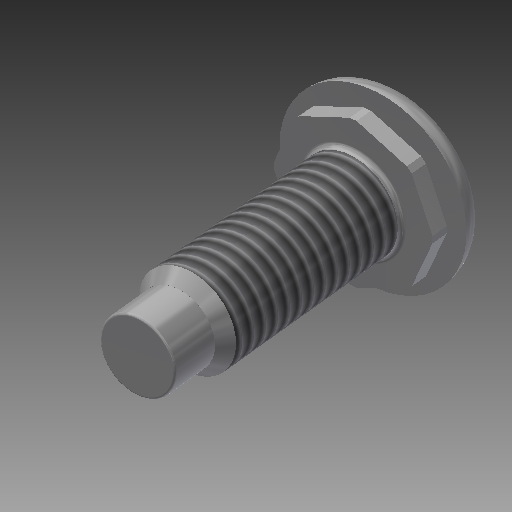
# Autodesk Inventor part: 314-10
Saved by Autodesk Inventor 2019 (Build 230136000, 136)
## iProperties
Company: Autodesk Inc.
Created: 2007-10-17
Part Number: 314-10
Document SubType Name: Modeling
Designer: Autodesk Inc.
Density: 7.85 g/cm^3
Mass: 23.0419 g
Surface Area: 17.262 cm^2
Volume: 2.93528 cm^3
Material: Steel, Mild
Description: DR342 M12 X 14
Appearance: Steel
Component Category: Fasteners
Author: Inventor
Autodesk Inventor part; units mm, degrees
ref_plane "YZ Plane" through (0, 0, 0) normal (1, 0, 0) x (0, 1, 0)
ref_plane "Work Plane1" through (2733.5993, 510.3823, 544.9206) normal (0.1045285, 0, 0.9945219) x (0.0000001, 1, 0)
sketch "Sketch1" plane through (2733.5993, 510.3823, 544.9206) normal (0.1045285, 0, 0.9945219) x (0.0000001, 1, 0)
  circle A0 centre (0, 3.6) radius 3.85
  line L0 (-510.3825, -1.79) -> (-510.3825, 8.99) projected
  line L1 (-5.3902, 2661.6646) -> (5.3898, 2661.6646) projected
  line L2 (-510.3824, 8.99) -> (-510.3824, -1.79) projected
  dimension "d0" = 7.7
  dimension "d1" = 510.3825
  dimension "d2" = 2658.0646
  constraints: 1 centre point
  measures "d0" diameter of A0
  measures "d1" distance from line of L0 A0.centre
  measures "d2" distance from line of L1 A0.centre
extrude "Extrusion1" add sketch "Sketch1" against normal blind 5
sketch "Sketch2" plane through (2729.4964, 510.3823, 540.3243) normal (-0.1045285, 0, -0.9945219) x (-0.9945219, 0, 0.1045285)
  circle A0 centre (0, 0) radius 3.85 projected
  circle A1 centre (0, 0) radius 4.9459
  dimension "d5" = 9.8917
  constraints: 1 centre point, 1 coincident
  measures "d5" diameter of A1
extrude "Extrusion2" add sketch "Sketch2" along normal blind 22.08 contours A0 | A1
sketch "Sketch3" plane through (2727.1884, 510.3823, 518.3653) normal (-0.1045285, 0, -0.9945219) x (-0.9945219, 0, 0.1045285)
  circle A0 centre (0, 0) radius 4.9459 projected
  line L0 (0, -8.1991) -> (-5.7976, -5.7977)
  line L1 (-5.7976, -5.7977) -> (-8.1991, 0)
  line L2 (-8.1991, 0) -> (-5.7977, 5.7976)
  line L3 (-5.7977, 5.7976) -> (0, 8.1991)
  line L4 (0, 8.1991) -> (5.7976, 5.7977)
  line L5 (5.7976, 5.7977) -> (8.1991, 0)
  line L6 (8.1991, 0) -> (5.7977, -5.7976)
  line L7 (5.7977, -5.7976) -> (0, -8.1991)
  line L8 (-12.0322, -510.3825) -> (14.7999, -510.3825) projected
  line L9 (2658.0646, -11.4788) -> (2658.0646, 11.4788) projected
  line L10 (14.7999, -510.3823) -> (-12.0323, -510.3823) projected
  dimension "d8" = 5.7976
  dimension "d9" = 2.4015
  constraints: 16 end point, 1 coincident, 17 other
  measures "d8" horizontal distance of L0.start L0.end
  measures "d9" vertical distance of L0.start L0.end
extrude "Extrusion3" add sketch "Sketch3" along normal blind 1.8 contours A0 | L0 L1 L2 L3 L4 L5 L6 L7
sketch "Sketch4" plane through (2727.0002, 510.3823, 516.5751) normal (-0.1045285, 0, -0.9945219) x (-0.9945219, 0, 0.1045285)
  circle A0 centre (0, 0) radius 6.3211
  line L0 (-12.2942, -510.3825) -> (15.0619, -510.3825) projected
  line L1 (2658.0646, -11.4788) -> (2658.0646, 11.4788) projected
  line L2 (15.0619, -510.3823) -> (-12.2942, -510.3823) projected
  dimension "d12" = 12.6421
  dimension "d14" = 510.3823
  dimension "d15" = 2658.0646
  constraints: 1 centre point
  measures "d12" diameter of A0
  measures "d14" distance from line of L2 A0.centre
  measures "d15" distance from line of L1 A0.centre
extrude "Extrusion4" add sketch "Sketch4" along normal blind 0.7
sketch "Sketch5" plane through (2726.927, 510.3823, 515.879) normal (-0.1045285, 0, -0.9945219) x (-0.9945219, 0, 0.1045285)
  circle A0 centre (0, 0) radius 6.3211 projected
  circle A1 centre (0, 0) radius 9.5
  dimension "d18" = 19
  constraints: 1 centre point, 1 coincident
  measures "d18" diameter of A1
extrude "Extrusion5" add sketch "Sketch5" along normal blind 3 contours A0 | A1
fillet "Fillet1" radius 3 1 edges at (2736.0614, 510.3823, 511.9024)
fillet "Fillet1" radius 1 1 edges at (2733.2866, 510.3823, 515.9144)
fillet "Fillet1" radius 0.5 1 edges at (2732.1071, 510.3823, 517.8483)
fillet "Fillet1" radius 0.25 1 edges at (2730.019, 506.5323, 545.2969)
sketch "Sketch6" plane through (2726.6135, 510.3823, 512.8954) normal (-0.1045285, 0, -0.9945219) x (-0.9945219, 0, 0.1045285)
  circle A0 centre (0, 0) radius 6.5 projected
  circle A1 centre (0, 0) radius 5
  dimension "d25" = 10
  constraints: 1 centre point, 1 coincident
  measures "d25" diameter of A1
extrude "Extrusion6" cut sketch "Sketch6" against normal blind 2 contours A1
fillet "Fillet2" radius 0.5 1 edges at (2731.7953, 510.3823, 514.3638)
chamfer "Chamfer2" distance 0.3766 angle 45 1 edges at (2727.0943, 502.1832, 517.4702)
chamfer "Chamfer3" distance 0.3766 angle 45 1 edges at (2732.8602, 504.5847, 516.8642)
chamfer "Chamfer4" distance 0.3766 angle 45 1 edges at (2735.2485, 510.3823, 516.6132)
chamfer "Chamfer5" distance 0.3766 angle 45 1 edges at (2732.8602, 516.18, 516.8642)
chamfer "Chamfer6" distance 0.3766 angle 45 1 edges at (2727.0943, 518.5815, 517.4702)
chamfer "Chamfer7" distance 0.3766 angle 45 1 edges at (2721.3284, 516.18, 518.0762)
chamfer "Chamfer8" distance 0.3766 angle 45 1 edges at (2718.9401, 510.3824, 518.3272)
chamfer "Chamfer9" distance 0.3766 angle 45 1 edges at (2721.3284, 504.5847, 518.0762)
ref_plane "Work Plane3" through (2730.0713, 509.1816, 518.0623) normal (0.3805886, 0.9238789, -0.0400015) x (-0.9188178, 0.382685, 0.0965716)
ref_plane "Work Plane2" through (2732.9543, 516.18, 517.7593) normal (0.3805886, 0.9238789, -0.0400015) x (-0.9188178, 0.382685, 0.0965716)
chamfer "Chamfer10" distance 1.095 distance2 1.298 1 edges at (2734.4151, 510.3823, 539.8073) measured on face at (2728.4119, 514.8065, 540.4383)
thread "Thread1" size "M10x1.5" class "6g" standard "ANSI Metric M Profile" full length
body "Solid1"
